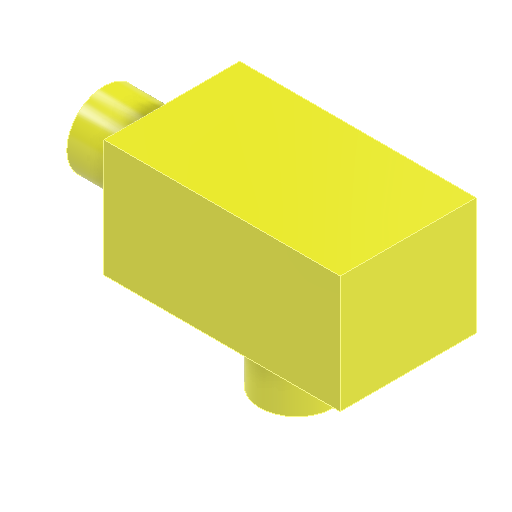
# Autodesk Inventor part: aux_L
Saved by Autodesk Inventor 2022 (Build 260153000, 153)
## iProperties
Created: 2021-04-23
Part Number: aux_L
Material: Generic
Document SubType Name: Modeling
Designer: nnico
Density: 1 g/cm^3
Appearance: Yellow
Author: nnico
Autodesk Inventor part; units mm, degrees
ref_plane "YZ Plane" through (0, 0, 0) normal (1, 0, 0) x (0, 1, 0)
ref_plane "XZ Plane" through (0, 0, 0) normal (0, 1, 0) x (-1, 0, 0)
ref_plane "XY Plane" through (0, 0, 0) normal (0, 0, 1) x (1, 0, 0)
sketch "Sketch1" plane through (0, 0, 0) normal (0, 0, 1) x (1, 0, 0)
  line L0 (-13.5, 24) -> (13.5, 24) construction
  line L1 (13.5, 24) -> (13.5, -24) construction
  line L2 (13.5, -24) -> (-13.5, -24) construction
  line L3 (-13.5, -24) -> (-13.5, 24) construction
  line L4 (-13.5, 0) -> (13.5, 0) construction
  line L5 (0, -24) -> (0, 24) construction
  circle A0 centre (0, 18.3) radius 2.75
  circle A1 centre (0, -18.3) radius 2.75
  line L6 (-60, 21.2) -> (-32, 21.2) construction
  line L7 (-32, 21.2) -> (-32, -25.8) construction
  line L8 (-32, -25.8) -> (-60, -25.8) construction
  line L9 (-60, -25.8) -> (-60, 21.2) construction
  line L10 (-46, 21.2) -> (-46, -25.8) construction
  line L11 (-60, -2.3) -> (-32, -2.3) construction
  circle A2 centre (-46, 15.7) radius 2.75
  circle A3 centre (-46, -20.3) radius 2.75
  circle A4 centre (46, 15.7) radius 2.75
  circle A5 centre (46, -20.3) radius 2.75
  line L12 (-82, 43.2) -> (82, 43.2)
  line L13 (82, 43.2) -> (82, -43.2)
  line L14 (82, -43.2) -> (-82, -43.2)
  line L15 (-82, -43.2) -> (-82, 43.2)
  point P0 (0, 0)
  point P1 (0, 0)
  dimension "d0" = 27
  dimension "d1" = 48
  dimension "d2" = 5.5
  dimension "d3" = 36.6
  dimension "d4" = 28
  dimension "d5" = 47
  dimension "d7" = 2.3
  dimension "d8" = 46
  dimension "d9" = 5.5
  dimension "d10" = 36
  dimension "d11" = 22
  dimension "d19" = 43.2
  constraints: 32 end point, 9 midpoint, 6 centre point, 6 parallel, 4 symmetric about line, 3 horizontal, 3 perpendicular, 2 point on line, 1 coincident, 6 other
  measures "d0" distance of L1.end L2.end
  measures "d1" distance of L0.end L1.end
  measures "d2" diameter of A0
  measures "d3" diameter of A0.centre L4
  measures "d4" distance of L7.end L8.end
  measures "d5" distance of L6.end L7.end
  measures "d7" distance from line of L11 L4.start
  measures "d8" horizontal distance of L5.end L10.start
  measures "d9" diameter of A2
  measures "d10" diameter of A2.centre L11
  measures "d11" distance from line of L15 L8.end
  measures "d19" distance from line of L12 L4.end
extrude "Extrusion1" add sketch "Sketch1" along normal blind 10
sketch "Sketch3" plane through (0, 0, 10) normal (0, 0, 1) x (1, 0, 0)
  line L0 (-82, 43.2) -> (-82, -43.2) projected
  line L1 (-82, -43.2) -> (82, -43.2) projected
  line L2 (-82, 43.2) -> (82, 43.2)
  line L3 (82, 43.2) -> (82, -43.2)
  line L4 (82, -43.2) -> (-82, -43.2)
  line L5 (-82, -43.2) -> (-82, 43.2)
  point P0 (0, 0)
  constraints: 8 end point, 2 parallel, 1 horizontal, 1 perpendicular
extrude "Extrusion3" add sketch "Sketch3" along normal blind 90
sketch "Sketch4" plane through (-82, -43.2, 0) normal (-1, 0, 0) x (0, 0, 1)
  line L0 (0, 86.4) -> (0, 0) projected
  line L1 (0, 0) -> (100, 0) projected
  line L2 (100, 86.4) -> (100, 0) projected
  line L3 (0, 86.4) -> (100, 86.4) projected
  point P0 (0, 43.2)
extrude "Extrusion4" add sketch "Sketch4" along normal blind 10
sketch "Sketch5" plane through (-92, -43.2, 0) normal (-1, 0, 0) x (0, 0, 1)
  line L0 (0, 43.2) -> (100, 43.2) construction
  line L1 (100, 0) -> (100, 86.4) construction
  line L2 (0, 86.4) -> (100, 86.4) construction
  line L3 (50, 86.4) -> (50, 0) construction
  line L4 (0, 0) -> (100, 0) construction
  circle A0 centre (50, 43.2) radius 27.305
  dimension "d22" = 54.61
  constraints: 4 end point, 4 midpoint, 1 centre point
  measures "d22" diameter of A0
extrude "Extrusion5" add sketch "Sketch5" along normal blind 50
sketch "Sketch6" plane through (82, -43.2, 0) normal (0, -1, 0) x (1, 0, 0)
  line L0 (0, 0) -> (0, 100) construction
  line L1 (0, 50) -> (-174, 50) construction
  line L2 (-174, 100) -> (-174, 0) construction
  line L3 (-82, 0) -> (-82, 100) construction
  line L4 (0, 100) -> (-174, 100) construction
  circle A0 centre (-82, 50) radius 27.305
  dimension "d25" = 54.61
  constraints: 4 end point, 3 midpoint, 1 centre point, 1 perpendicular, 1 point on line
  measures "d25" diameter of A0
extrude "Extrusion6" add sketch "Sketch6" along normal blind 50
body "Solid1"
